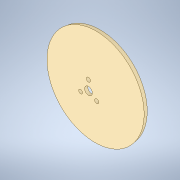
# Autodesk Inventor part: Бортик конусной катушки
Saved by Autodesk Inventor 2021.1 (Build 251245010, 245A)
## iProperties
Created: 2026-04-13
Part Number: Бортик конусной катушки
Material: Типовые
Document SubType Name: Modeling
Designer: Андрей Тарасов
Density: 1 g/cm^3
Appearance: По умолчанию
Author: Андрей Тарасов
Autodesk Inventor part; units mm, degrees
ref_plane "YZ Plane" through (0, 0, 0) normal (1, 0, 0) x (0, 1, 0)
ref_plane "XZ Plane" through (0, 0, 0) normal (0, 1, 0) x (-1, 0, 0)
ref_plane "XY Plane" through (0, 0, 0) normal (0, 0, 1) x (1, 0, 0)
sketch "Эскиз1" plane through (0, 0, 0) normal (0, 0, 1) x (1, 0, 0)
  circle A0 centre (0, 0) radius 5
  circle A1 centre (0, 0) radius 60
  line L0 (0, -84) -> (0, 84) construction
  circle A2 centre (0, 0) radius 20.7 construction
  circle A3 centre (0, 12) radius 2.6
  line L1 (-84, 0) -> (84, 0) construction
  circle A4 centre (-10.3923, -6) radius 2.6
  circle A5 centre (10.3923, -6) radius 2.6
  dimension "d0" = 10
  dimension "d1" = 120
  dimension "d4" = 41.4
  dimension "d5" = 5.2
  dimension "d6" = 12
  dimension "d9" = 360
  constraints: 6 centre point, 3 coincident, 1 point on line, 7 other
  measures "d0" diameter of A0
  measures "d1" diameter of A1
  measures "d4" diameter of A2
  measures "d5" diameter of A3
  measures "d6" distance from line of L1 A3.centre
extrude "Выдавливание1" add sketch "Эскиз1" along normal blind 4
